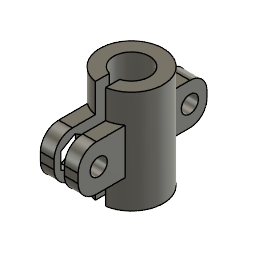
Soporte superior camara (Autodesk Fusion 360 design; units mm, degrees)
part number: 2026-03-01-15-50-44-242
Autodesk Fusion 360 part; units mm, degrees
sketch "Boceto1" plane through (0, 0, 0) normal (0, 1, 0) x (1, 0, 0)
  line L0 (0, 0) -> (0, -5.15)
  line L1 (1.5, -4.979) -> (1.5, -9.0769)
  line L2 (-1.5, -4.979) -> (-1.5, -9.0769)
  arc A0 (1.5, -4.979) -> (-1.5, -4.979) centre (0, 0) ccw
  arc A1 (1.5, -9.0769) -> (-1.5, -9.0769) centre (0, 0) ccw
  dimension "d1" = 10.4
  dimension "d2" = 4
  dimension "d3" = 1.5
  dimension "d4" = 1.5
  constraint coincident L0.start A0.centre
  constraint vertical L0
  constraint vertical L1
  constraint vertical L2
  measures "d1" diameter of A0
  measures "d2" distance of A0 A1
  measures "d3" distance of L0 L1
  measures "d4" distance of L0 L2
extrude "Extruir1" add sketch "Boceto1" along normal blind 30 makes body 1
sketch "Boceto2" plane through (1.5, 0, 0) normal (-1, 0, 0) x (0, 0, 1)
  line L0 (4.979, 0) -> (9.0769, 0)
  line L1 (9.0769, 0) -> (9.0769, 30)
  line L2 (9.0769, 30) -> (4.979, 30)
  line L3 (4.979, 30) -> (4.979, 0)
  line L4 (9.0769, 0) -> (9.0769, 30)
  line L5 (9.0769, 15) -> (18, 15) construction
  line L6 (9.0769, 21.6188) -> (15.7482, 21.6188)
  line L7 (9.0769, 8.3812) -> (15.7482, 8.3812)
  line L8 (15.0769, 19.6188) -> (11.0769, 17.3094)
  line L9 (11.0769, 17.3094) -> (11.0769, 12.6906)
  line L10 (11.0769, 12.6906) -> (15.0769, 10.3812)
  line L11 (15.0769, 10.3812) -> (19.0769, 12.6906)
  line L12 (19.0769, 12.6906) -> (19.0769, 17.3094)
  line L13 (19.0769, 17.3094) -> (15.0769, 19.6188)
  line L14 (21.0769, 16.2902) -> (21.0769, 13.7098)
  arc A0 (21.0769, 16.2902) -> (15.7482, 21.6188) centre (15.7482, 16.2902) ccw
  arc A1 (15.7482, 8.3812) -> (21.0769, 13.7098) centre (15.7482, 13.7098) ccw
  point P0 (15.0769, 15)
  dimension "d22" = 8
  dimension "d23" = 2
  dimension "d24" = 2
  dimension "d25" = 2
  dimension "d26" = 2
  constraint midpoint L4 L5.start
  constraint perpendicular L4 L5
  constraint coincident L4 L6.start
  constraint perpendicular L4 L6
  constraint coincident L4 L7.start
  constraint coincident L5 P0
  constraint vertical L14
  constraint tangent L6 A0
  constraint tangent L14 A0
  constraint symmetric L5 L6.end L7.end
  constraint symmetric L5 L14.start L14.end
  constraint symmetric L5 A0 A1
  measures "d22" distance of L8 L11
  measures "d23" distance of L4 L9
  measures "d24" distance of L7 L10.end
  measures "d25" distance of L6 L8.start
  measures "d26" distance of L12 L14
extrude "Extruir2" add sketch "Boceto2" against normal blind 4 separate body contours L1 L4 L6 L7 L14 A0 A1 | L8 L9 L10 L11 L12 L13 makes body 2
sketch "Boceto3" plane through (0, 0, 9.0769) normal (0, 0, -1) x (-1, 0, 0)
  line L0 (-1.5, 8.3812) -> (-1.5, 21.6188)
  line L1 (-1.5, 21.6188) -> (-5.5, 21.6188)
  line L2 (-5.5, 21.6188) -> (-5.5, 8.3812)
  line L3 (-5.5, 8.3812) -> (-1.5, 8.3812)
  line L4 (9.2, 0) -> (-9.2, 0)
  line L5 (1.5, 0) -> (1.5, 30)
  line L6 (9.2, 30) -> (-9.2, 30)
  line L7 (-1.5, 30) -> (-1.5, 0)
extrude "Extruir3" add sketch "Boceto3" along normal up to surface contours L0 L1 L2 L3 L7 end surface at (-2.3921, 20, 8.8836) on bodies 1 bodies 1 2
sketch "Boceto4" plane through (5.5, 0, 0) normal (1, 0, 0) x (0, 0, -1)
  line L0 (-15.7482, 8.3812) -> (-7.375, 8.3812)
  line L1 (-7.375, 8.3812) -> (-7.375, 21.6188)
  line L2 (-7.375, 21.6188) -> (-15.7482, 21.6188)
  arc A0 (-15.7482, 21.6188) -> (-21.0769, 16.2902) centre (-15.7482, 16.2902) ccw
  line L3 (-21.0769, 16.2902) -> (-21.0769, 13.7098)
  arc A1 (-21.0769, 13.7098) -> (-15.7482, 8.3812) centre (-15.7482, 13.7098) ccw
  circle A2 centre (-15.0769, 15) radius 2.5
  point P0 (-24.2638, 15)
  point P1 (-21.2636, 15.0299)
  dimension "d27" = 5
  dimension "d28" = 6
  measures "d27" diameter of A2
  measures "d28" horizontal distance of L3.end A2.centre
extrude "Extruir4" cut sketch "Boceto4" against normal through all contours A2 bodies 1
ref_plane "PlanoDeObra1" through (0, 15, 7.0279) normal (1, 0, 0) x (0, 0, -1)
mirror "Simetría1" about plane through (0, 15, 7.0279) normal (1, 0, 0) of bodies 1 merged
sketch "Boceto5" plane through (-5.5, 0, 0) normal (-1, 0, 0) x (0, 0, 1)
  line L0 (7.375, 8.3812) -> (15.7482, 8.3812)
  line L1 (15.7482, 21.6188) -> (7.375, 21.6188)
  line L2 (7.375, 21.6188) -> (7.375, 8.3812)
  line L3 (15, 19.7343) -> (10.9, 17.3671)
  line L4 (10.9, 17.3671) -> (10.9, 12.6329)
  line L5 (10.9, 12.6329) -> (15, 10.2657)
  line L6 (15, 10.2657) -> (19.1, 12.6329)
  line L7 (19.1, 12.6329) -> (19.1, 17.3671)
  line L8 (19.1, 17.3671) -> (15, 19.7343)
  point P0 (15, 15)
  dimension "d29" = 8.2
  measures "d29" distance of L3 L6
extrude "Extruir5" cut sketch "Boceto5" against normal up to surface (4 mm away) bodies 1
sketch "Boceto6" plane through (-5.5, 0, 0) normal (-1, 0, 0) x (0, 0, 1)
  line L0 (19.1, 12.6329) -> (15, 10.2657)
  line L1 (15, 10.2657) -> (10.9, 12.6329)
  line L2 (10.9, 12.6329) -> (10.9, 17.3671)
  line L3 (10.9, 17.3671) -> (15, 19.7343)
  line L4 (15, 19.7343) -> (19.1, 17.3671)
  line L5 (19.1, 17.3671) -> (19.1, 12.6329)
  line L6 (15.7482, 21.6188) -> (7.375, 21.6188)
  line L7 (7.375, 21.6188) -> (7.375, 8.3812)
  line L8 (7.375, 8.3812) -> (15.7482, 8.3812)
  arc A0 (15.7482, 8.3812) -> (21.0769, 13.7098) centre (15.7482, 13.7098) ccw
  line L9 (21.0769, 13.7098) -> (21.0769, 16.2902)
  arc A1 (21.0769, 16.2902) -> (15.7482, 21.6188) centre (15.7482, 16.2902) ccw
sketch "Boceto10" plane through (0, 0, 0) normal (1, 0, 0) x (0, 0, -1)
  line L0 (9, 21) -> (12, 21)
  line L1 (17, 16) -> (17, 14)
  line L2 (12, 9) -> (9, 9)
  line L3 (9, 9) -> (9, 21)
  line L4 (9.2, 0) -> (-9.0769, 0)
  arc A0 (17, 16) -> (12, 21) centre (12, 16) ccw
  arc A1 (12, 9) -> (17, 14) centre (12, 14) ccw
  circle A2 centre (13, 15) radius 2.5
  point P0 (17, 9)
  dimension "d42" = 12
  dimension "d43" = 8
  dimension "d44" = 9
  dimension "d45" = 5
  dimension "d46" = 5
  dimension "d47" = 4
  constraint horizontal L0
  constraint vertical L1
  constraint horizontal L2
  constraint vertical L3
  constraint tangent L0 A0
  constraint tangent L1 A0
  constraint coincident P0 L2
  constraint coincident P0 L1
  constraint tangent L2 A1
  constraint tangent L1 A1
  constraint equal A0 A1
  measures "d42" distance of L0 L2
  measures "d43" distance of P0 L2.end
  measures "d44" distance of L2 L4
  measures "d45" radius of A0
  measures "d46" diameter of A2
  measures "d47" distance of L3 A2.centre
sketch "Boceto11" plane through (0, 0, 0) normal (1, 0, 0) x (0, 0, -1)
  line L0 (9, 21) -> (9, 9)
  line L1 (19, 16) -> (19, 14)
  line L2 (9, 21) -> (14, 21)
  line L3 (9, 9) -> (14, 9)
  line L4 (9, 9) -> (9, 21)
  arc A0 (19, 16) -> (14, 21) centre (14, 16) ccw
  arc A1 (14, 9) -> (19, 14) centre (14, 14) ccw
  line L5 (9, 21) -> (9, 9)
  circle A2 centre (14, 15) radius 2.5
  line L6 (9.2, 0) -> (-9.0769, 0)
  dimension "d48" = 10
  dimension "d49" = 5
  dimension "d50" = 5
  dimension "d51" = 5
  dimension "d52" = 12
  dimension "d53" = 9
  dimension "d54" = 6
  constraint vertical L0
  constraint vertical L1
  constraint perpendicular L0 L2
  constraint perpendicular L0 L3
  constraint tangent L2 A0
  constraint tangent L3 A1
  constraint tangent L1 A1
  constraint equal A0 A1
  measures "d48" distance of L1 L4
  measures "d49" radius of A0
  measures "d50" diameter of A2
  measures "d51" distance of L5 A2.centre
  measures "d52" distance of L2 L3
  measures "d53" distance of L3 L6
  measures "d54" distance of L3 A2.centre
extrude "Extruir8" cut sketch "Boceto11" along normal mid plane 8 bodies 1
extrude "Extruir9" add sketch "Boceto11" along normal mid plane 6 bodies 1
extrude "Extruir10" add 1 faces at (-2.636, 17, -9) along direction (0, 0, 1) up to surface end surface at (6.5616, 20, -6.4486) on bodies 1 bodies 1
extrude "Extruir11" add 1 faces at (2.2719, 17, -9) along direction (0, 0, 1) up to surface end surface at (6.5616, 20, -6.4486) on bodies 1 bodies 1
